Autodesk Fusion 360 part; units mm, degrees
(part 7 of 7)
  spline S37 degree 5 poles (10.9042, -14.0526) (10.9032, -14.0442) (10.9013, -14.0274) (10.8983, -14.0021) (10.8942, -13.9685) (10.889, -13.9266) (10.8835, -13.8847) (10.8779, -13.8429) (10.8721, -13.8013) (10.8661, -13.7597) (10.8598, -13.7182) (10.8535, -13.6768) (10.8469, -13.6355) (10.8401, -13.5943) (10.8331, -13.5531) (10.8259, -13.5121) (10.8186, -13.4712) (10.811, -13.4304) (10.8033, -13.3896) (10.7953, -13.349) (10.7872, -13.3085) (10.7788, -13.2681) (10.7703, -13.2278) (10.7615, -13.1876) (10.7526, -13.1475) (10.7434, -13.1075) (10.7341, -13.0676) (10.7245, -13.0279) (10.7147, -12.9883) (10.7048, -12.9487) (10.6946, -12.9093) (10.6842, -12.8701) (10.6736, -12.8309) (10.6628, -12.7919) (10.6517, -12.753) (10.6405, -12.7142) (10.629, -12.6755) (10.6174, -12.637) (10.6055, -12.5987) (10.5933, -12.5604) (10.581, -12.5223) (10.5684, -12.4844) (10.5556, -12.4466) (10.5426, -12.4089) (10.5293, -12.3714) (10.5158, -12.334) (10.502, -12.2968) (10.4881, -12.2598) (10.4738, -12.2229) (10.4594, -12.1862) (10.4446, -12.1497) (10.4296, -12.1133) (10.4144, -12.0772) (10.3988, -12.0412) (10.383, -12.0054) (10.3669, -11.9698) (10.3505, -11.9344) (10.3339, -11.8992) (10.3171, -11.8642) (10.2999, -11.8294) (10.2824, -11.7948) (10.2645, -11.7605) (10.2462, -11.7266) (10.2274, -11.693) (10.2082, -11.6597) (10.1888, -11.6266) (10.1691, -11.5937) (10.1493, -11.561) (10.1291, -11.5285) (10.1084, -11.4965) (10.0869, -11.4651) (10.0686, -11.4408) (10.0543, -11.4231) (10.0444, -11.4116) (10.0394, -11.4059) knots -1 -1 -1 -1 -1 -1 -0.98571429 -0.97142857 -0.95714286 -0.94285714 -0.92857143 -0.91428571 -0.9 -0.88571429 -0.87142857 -0.85714286 -0.84285714 -0.82857143 -0.81428571 -0.8 -0.78571429 -0.77142857 -0.75714286 -0.74285714 -0.72857143 -0.71428571 -0.7 -0.68571429 -0.67142857 -0.65714286 -0.64285714 -0.62857143 -0.61428571 -0.6 -0.58571429 -0.57142857 -0.55714286 -0.54285714 -0.52857143 -0.51428571 -0.5 -0.48571429 -0.47142857 -0.45714286 -0.44285714 -0.42857143 -0.41428571 -0.4 -0.38571429 -0.37142857 -0.35714286 -0.34285714 -0.32857143 -0.31428571 -0.3 -0.28571429 -0.27142857 -0.25714286 -0.24285714 -0.22857143 -0.21428571 -0.2 -0.18571429 -0.17142857 -0.15714286 -0.14285714 -0.12857143 -0.11428571 -0.1 -0.08571429 -0.07142857 -0.05714286 -0.04285714 -0.02857143 -0.01428571 0 0 0 0 0 0
  line L37 (10.0394, -11.4059) -> (9.6289, -10.9387)
  arc A74 (9.657, -10.3818) -> (9.6289, -10.9387) centre (9.9294, -10.6747) ccw
  arc A75 (9.657, -10.3818) -> (10.3818, -9.657) centre (0, 0) ccw
  arc A76 (10.9387, -9.6289) -> (10.3818, -9.657) centre (10.6747, -9.9294) ccw
  line L38 (10.9387, -9.6289) -> (11.4059, -10.0394)
  spline S38 degree 5 poles (11.4059, -10.0394) (11.4116, -10.0444) (11.4231, -10.0543) (11.4408, -10.0686) (11.4651, -10.0869) (11.4965, -10.1084) (11.5285, -10.1291) (11.561, -10.1493) (11.5937, -10.1691) (11.6266, -10.1888) (11.6597, -10.2082) (11.693, -10.2274) (11.7266, -10.2462) (11.7605, -10.2645) (11.7948, -10.2824) (11.8294, -10.2999) (11.8642, -10.3171) (11.8992, -10.3339) (11.9344, -10.3505) (11.9698, -10.3669) (12.0054, -10.383) (12.0412, -10.3988) (12.0772, -10.4144) (12.1133, -10.4296) (12.1497, -10.4446) (12.1862, -10.4594) (12.2229, -10.4738) (12.2598, -10.4881) (12.2968, -10.502) (12.334, -10.5158) (12.3714, -10.5293) (12.4089, -10.5426) (12.4466, -10.5556) (12.4844, -10.5684) (12.5223, -10.581) (12.5604, -10.5933) (12.5987, -10.6055) (12.637, -10.6174) (12.6755, -10.629) (12.7142, -10.6405) (12.753, -10.6517) (12.7919, -10.6628) (12.8309, -10.6736) (12.8701, -10.6842) (12.9093, -10.6946) (12.9487, -10.7048) (12.9883, -10.7147) (13.0279, -10.7245) (13.0676, -10.7341) (13.1075, -10.7434) (13.1475, -10.7526) (13.1876, -10.7615) (13.2278, -10.7703) (13.2681, -10.7788) (13.3085, -10.7872) (13.349, -10.7953) (13.3896, -10.8033) (13.4304, -10.811) (13.4712, -10.8186) (13.5121, -10.8259) (13.5531, -10.8331) (13.5943, -10.8401) (13.6355, -10.8469) (13.6768, -10.8535) (13.7182, -10.8598) (13.7597, -10.8661) (13.8013, -10.8721) (13.8429, -10.8779) (13.8847, -10.8835) (13.9266, -10.889) (13.9685, -10.8942) (14.0021, -10.8983) (14.0274, -10.9013) (14.0442, -10.9032) (14.0526, -10.9042) knots 0 0 0 0 0 0 0.01428571 0.02857143 0.04285714 0.05714286 0.07142857 0.08571429 0.1 0.11428571 0.12857143 0.14285714 0.15714286 0.17142857 0.18571429 0.2 0.21428571 0.22857143 0.24285714 0.25714286 0.27142857 0.28571429 0.3 0.31428571 0.32857143 0.34285714 0.35714286 0.37142857 0.38571429 0.4 0.41428571 0.42857143 0.44285714 0.45714286 0.47142857 0.48571429 0.5 0.51428571 0.52857143 0.54285714 0.55714286 0.57142857 0.58571429 0.6 0.61428571 0.62857143 0.64285714 0.65714286 0.67142857 0.68571429 0.7 0.71428571 0.72857143 0.74285714 0.75714286 0.77142857 0.78571429 0.8 0.81428571 0.82857143 0.84285714 0.85714286 0.87142857 0.88571429 0.9 0.91428571 0.92857143 0.94285714 0.95714286 0.97142857 0.98571429 1 1 1 1 1 1
  arc A77 (14.0526, -10.9042) -> (14.713, -9.9953) centre (0, 0) ccw
  spline S39 degree 5 poles (14.713, -9.9953) (14.7095, -9.9876) (14.7024, -9.9721) (14.6918, -9.949) (14.6775, -9.9183) (14.6596, -9.8801) (14.6415, -9.8419) (14.6232, -9.804) (14.6048, -9.7661) (14.5862, -9.7284) (14.5675, -9.6909) (14.5486, -9.6535) (14.5296, -9.6162) (14.5104, -9.5791) (14.491, -9.5422) (14.4716, -9.5054) (14.4519, -9.4687) (14.4321, -9.4323) (14.4121, -9.3959) (14.392, -9.3597) (14.3718, -9.3237) (14.3513, -9.2879) (14.3307, -9.2522) (14.31, -9.2166) (14.2891, -9.1813) (14.268, -9.1461) (14.2468, -9.1111) (14.2254, -9.0762) (14.2039, -9.0415) (14.1822, -9.007) (14.1604, -8.9727) (14.1383, -8.9386) (14.1162, -8.9046) (14.0938, -8.8708) (14.0713, -8.8372) (14.0486, -8.8038) (14.0258, -8.7706) (14.0028, -8.7376) (13.9796, -8.7048) (13.9562, -8.6721) (13.9327, -8.6397) (13.909, -8.6075) (13.8852, -8.5755) (13.8611, -8.5437) (13.8369, -8.5122) (13.8125, -8.4808) (13.788, -8.4497) (13.7632, -8.4188) (13.7383, -8.3881) (13.7132, -8.3576) (13.6879, -8.3274) (13.6624, -8.2975) (13.6367, -8.2678) (13.6108, -8.2384) (13.5847, -8.2093) (13.5584, -8.1805) (13.5319, -8.1518) (13.5052, -8.1235) (13.4784, -8.0953) (13.4513, -8.0675) (13.424, -8.0401) (13.3963, -8.013) (13.3684, -7.9864) (13.3402, -7.9603) (13.3116, -7.9346) (13.2829, -7.9091) (13.2541, -7.8839) (13.2251, -7.8589) (13.1959, -7.8342) (13.1663, -7.8101) (13.1361, -7.787) (13.1112, -7.7695) (13.0921, -7.7571) (13.0791, -7.7492) (13.0726, -7.7453) knots -1 -1 -1 -1 -1 -1 -0.98571429 -0.97142857 -0.95714286 -0.94285714 -0.92857143 -0.91428571 -0.9 -0.88571429 -0.87142857 -0.85714286 -0.84285714 -0.82857143 -0.81428571 -0.8 -0.78571429 -0.77142857 -0.75714286 -0.74285714 -0.72857143 -0.71428571 -0.7 -0.68571429 -0.67142857 -0.65714286 -0.64285714 -0.62857143 -0.61428571 -0.6 -0.58571429 -0.57142857 -0.55714286 -0.54285714 -0.52857143 -0.51428571 -0.5 -0.48571429 -0.47142857 -0.45714286 -0.44285714 -0.42857143 -0.41428571 -0.4 -0.38571429 -0.37142857 -0.35714286 -0.34285714 -0.32857143 -0.31428571 -0.3 -0.28571429 -0.27142857 -0.25714286 -0.24285714 -0.22857143 -0.21428571 -0.2 -0.18571429 -0.17142857 -0.15714286 -0.14285714 -0.12857143 -0.11428571 -0.1 -0.08571429 -0.07142857 -0.05714286 -0.04285714 -0.02857143 -0.01428571 0 0 0 0 0 0
  line L39 (13.0726, -7.7453) -> (12.5379, -7.4278)
  arc A78 (12.3925, -6.8895) -> (12.5379, -7.4278) centre (12.7421, -7.0839) ccw
  arc A79 (12.3925, -6.8895) -> (12.8578, -5.9762) centre (0, 0) ccw
  circle A80 centre (0, 0) radius 3.5
  circle A81 centre (0, 0) radius 25
  dimension "d42" = 50
  constraint coincident A1.centre A3.centre
  measures "d42" diameter of A81
extrude "Extrude16" add sketch "Sketch10" along normal blind 2 contours A0 L0 S0 A1 S1 L1 A2 A3 A4 L2 S2 A5 S3 L3 A6 A7 A8 L4 S4 A9 S5 L5 A10 A11 A12 L6 S6 A13 S7 L7 A14 A15 A16 L8 S8 A17 S9 L9 A18 A19 A20 L10 S10 A21 S11 L11 A22 A23 A24 L12 S12 A25 S13 L13 A26 A27 A28 L14 S14 A29 S15 L15 A30 A31 A32 L16 S16 A33 S17 L17 A34 A35 A36 L18 S18 A37 S19 L19 A38 A39 A40 L20 S20 A41 S21 L21 A42 A43 A44 L22 S22 A45 S23 L23 A46 A47 A48 L24 S24 A49 S25 L25 A50 A51 A52 L26 S26 A53 S27 L27 A54 A55 A56 L28 S28 A57 S29 L29 A58 A59 A60 L30 S30 A61 S31 L31 A62 A63 A64 L32 S32 A65 S33 L33 A66 A67 A68 L34 S34 A69 S35 L35 A70 A71 A72 L36 S36 A73 S37 L37 A74 A75 A76 L38 S38 A77 S39 L39 A78 A79 | A81 in component "Spur Gear (20 teeth)"
component "Spur Gear (20 teeth)" placed x (1, 0, 0) y (0, 1, 0) z (0, 0, 1) at (0, 0, 0)
